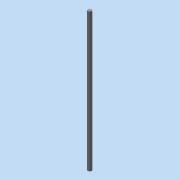
# Autodesk Inventor part: Star Axle
Saved by Autodesk Inventor 2015 (Build 190159000, 159)
## iProperties
Created: 2014-09-21
Part Number: Star Axle
Material: Generic
Document SubType Name: Modeling
Designer: Kris
Density: 1 g/cm^3
Appearance: Default
Author: Kris
Autodesk Inventor part; units mm, degrees
ref_plane "YZ Plane" through (0, 0, 0) normal (1, 0, 0) x (0, 1, 0)
ref_plane "XZ Plane" through (0, 0, 0) normal (0, 1, 0) x (-1, 0, 0)
ref_plane "XY Plane" through (0, 0, 0) normal (0, 0, 1) x (1, 0, 0)
sketch "Sketch1" plane through (0, 0, 0) normal (0, 1, 0) x (-1, 0, 0)
  line L0 (0, -2.5) -> (-2.3776, -0.7725)
  line L1 (-2.3776, -0.7725) -> (-1.4695, 2.0225)
  line L2 (-1.4695, 2.0225) -> (1.4695, 2.0225)
  line L3 (1.4695, 2.0225) -> (2.3776, -0.7725)
  line L4 (2.3776, -0.7725) -> (0, -2.5)
  point P0 (0, 0)
  point P1 (0, 0)
  point P2 (0, 0)
  constraints: 10 end point, 1 coincident, 11 other
extrude "Extrusion1" add sketch "Sketch1" along normal blind 177.8
body "Solid1"
